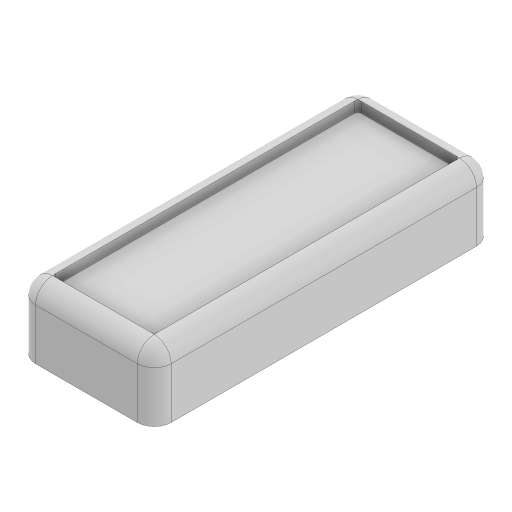
# Autodesk Inventor part: lcd screen
Saved by Autodesk Inventor 2024 (Build 280153000, 153)
## iProperties
Created: 2023-09-16
Part Number: lcd screen
Material: Generic
Document SubType Name: Modeling
Designer: draev
Density: 1 g/cm^3
Appearance: Default
Author: draev
Autodesk Inventor part; units mm, degrees
ref_plane "YZ Plane" through (0, 0, 0) normal (1, 0, 0) x (0, 1, 0)
ref_plane "XZ Plane" through (0, 0, 0) normal (0, 1, 0) x (-1, 0, 0)
ref_plane "XY Plane" through (0, 0, 0) normal (0, 0, 1) x (1, 0, 0)
sketch "Sketch1" plane through (0, 0, 0) normal (0, 1, 0) x (-1, 0, 0)
  line L0 (0, 0) -> (80, 0)
  line L1 (80, 0) -> (80, 200)
  line L2 (80, 200) -> (0, 200)
  line L3 (0, 200) -> (0, 0)
  dimension "d0" = 80
  dimension "d1" = 200
  constraints: 8 end point, 2 parallel, 1 horizontal, 1 perpendicular
  measures "d0" distance of L2.end L1.end
  measures "d1" distance of L0.end L1.end
extrude "Extrusion1" add sketch "Sketch1" along normal blind 40
fillet "Fillet1" radius 10 8 edges at (0, 40, 100) (-40, 40, 200) (-80, 40, 100) (-40, 40, 0) (0, 20, 0) (0, 20, 200) (-80, 20, 200) (-80, 20, 0)
sketch "Sketch2" plane through (0, 40, 0) normal (0, 1, 0) x (1, 0, 0)
  line L0 (-68, -190) -> (-12, -190)
  line L1 (-10, -188) -> (-10, -12)
  line L2 (-12, -10) -> (-68, -10)
  line L3 (-70, -12) -> (-70, -188)
  line L4 (-70, -10) -> (-10, -10) projected
  line L5 (-10, -10) -> (-10, -190) projected
  arc A0 (-70, -188) -> (-68, -190) centre (-68, -188) ccw
  arc A1 (-68, -10) -> (-70, -12) centre (-68, -12) ccw
  arc A2 (-10, -12) -> (-12, -10) centre (-12, -12) ccw
  arc A3 (-12, -190) -> (-10, -188) centre (-12, -188) ccw
  point P0 (0, 0)
  point P1 (-70, -100)
  point P2 (-40, -10)
  dimension "d5" = 90
  dimension "d6" = 180
  dimension "d7" = 30
  dimension "d8" = 60
  dimension "d9" = 2
  constraints: 8 end point, 8 point on circle, 8 tangent, 4 centre point, 3 equal radius, 2 midpoint, 2 parallel, 1 horizontal, 1 perpendicular
  measures "d5" distance from line of L4 point (-70, -100)
  measures "d6" distance between parallel lines of L0 L2
  measures "d7" distance from line of L5 point (-40, -10)
  measures "d8" distance between parallel lines of L1 L3
  measures "d9" radius of A0
extrude "Extrusion2" cut sketch "Sketch2" against normal blind 6 contours A0 L3 A1 L2 A2 L1 A3 L0
body "Solid1"
